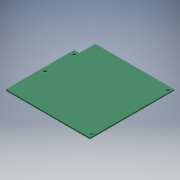
# Autodesk Inventor part: PCB
Saved by Autodesk Inventor 2017 (Build 210142000, 142)
## iProperties
Created: 2019-01-31
Part Number: PCB
Material: Generic
Document SubType Name: Modeling
Designer: Mitch
Density: 1 g/cm^3
Appearance: Smooth - Dark Sea Green
Author: Mitch
Autodesk Inventor part; units mm, degrees
ref_plane "YZ Plane" through (0, 0, 0) normal (1, 0, 0) x (0, 1, 0)
ref_plane "XZ Plane" through (0, 0, 0) normal (0, 1, 0) x (-1, 0, 0)
ref_plane "XY Plane" through (0, 0, 0) normal (0, 0, 1) x (1, 0, 0)
sketch "Sketch1" plane through (0, 0, 0) normal (0, 1, 0) x (-1, 0, 0)
  line L0 (0, 0) -> (104.14, 0)
  line L1 (104.14, 0) -> (104.14, -104.14)
  line L2 (104.14, -104.14) -> (0, -104.14)
  line L3 (0, -104.14) -> (0, 0)
  dimension "d0" = 104.14
  dimension "d1" = 104.14
  constraints: 8 end point, 2 parallel, 1 horizontal, 1 perpendicular
  measures "d0" distance of L1.end L2.end
  measures "d1" distance of L0.end L1.end
extrude "Extrusion1" add sketch "Sketch1" along normal blind 1.5748
hole "Hole1" at (-2.54, 1.5748, -5.08) direction (0, -1, 0) diameter 3.2766 depth 25.4 clearance for "Flat Head Machine Screw (82)" size "#4" standard "Ansi Unified Screw Threads"
hole "Hole2" at (-2.54, 1.5748, -99.06) direction (0, -1, 0) diameter 3.2766 depth 25.4 clearance for "Flat Head Machine Screw (82)" size "#4" standard "Ansi Unified Screw Threads"
sketch "Sketch3" plane through (0, 1.5748, 0) normal (0, 1, 0) x (1, 0, 0)
  line L0 (0, 104.14) -> (-104.14, 104.14) projected
  line L1 (-104.14, 104.14) -> (-97.5106, 104.14)
  line L2 (-97.5106, 104.14) -> (-97.5106, 84.328)
  line L3 (-97.5106, 84.328) -> (-104.14, 84.328)
  line L4 (-104.14, 84.328) -> (-104.14, 104.14)
  line L5 (-104.14, 0) -> (0, 0) projected
  dimension "d46" = 6.6294
  dimension "d47" = 84.328
  constraints: 8 end point, 2 parallel, 1 horizontal, 1 perpendicular
  measures "d46" distance of L2.end L3.end
  measures "d47" distance between parallel lines of L5 L3
extrude "Extrusion3" cut sketch "Sketch3" against normal blind 25.4
hole "Hole5" at (-99.06, 1.5748, -79.248) direction (0, -1, 0) diameter 3.2766 depth 25.4 clearance for "Flat Head Machine Screw (82)" size "#4" standard "Ansi Unified Screw Threads"
hole "Hole6" at (-99.06, 1.5748, -43.434) direction (0, -1, 0) diameter 3.2766 depth 25.4 clearance for "Flat Head Machine Screw (82)" size "#4" standard "Ansi Unified Screw Threads"
body "Solid1"
